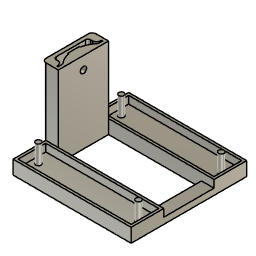
din_mount_cap_mcb_powerdist v2 (Autodesk Fusion 360 design; units mm, degrees)
Autodesk Fusion 360 part; units mm, degrees
note: some values were not read from the file. Set by a fixed rule: which sketch regions a step uses.
sketch "Sketch1" plane through (0, 0, 0) normal (0, 0, 1) x (1, 0, 0)
  line L0 (6.57, 33.77) -> (5.04, 33.77)
  line L1 (6.7574, 27.6038) -> (6.8807, 27.9464)
  arc A0 (5.5327, 24.59) -> (6.0311, 24.9915) centre (5.5327, 25.1) ccw
  arc A1 (10.1614, 33.4653) -> (6.8164, 27.7655) centre (24.5119, 21.2122) ccw
  line L2 (10.65, 34.79) -> (10.65, 37.85)
  line L3 (9.63, 3.17) -> (9.63, 2.15)
  arc A2 (6.0311, 15.0085) -> (6.8164, 12.2345) centre (28.9539, 20) ccw
  arc A3 (9.63, 3.17) -> (6.57, 6.23) centre (6.57, 3.17) ccw
  arc A4 (10.65, 5.21) -> (10.1614, 6.5347) centre (8.61, 5.21) ccw
  arc A5 (10.1614, 33.4653) -> (6.8164, 27.7655) centre (24.5119, 21.2122) ccw
  line L4 (5.1639, 24.59) -> (5.5327, 24.59)
  arc A6 (6.7574, 12.3962) -> (6.8164, 12.2345) centre (24.5119, 18.7878) ccw
  arc A7 (3, 8.27) -> (5.04, 6.23) centre (5.04, 8.27) ccw
  arc A8 (5.5327, 24.59) -> (6.0311, 24.9915) centre (5.5327, 25.1) ccw
  line L5 (11, 0) -> (11, 40)
  line L6 (0, 37) -> (0, 3)
  arc A9 (6.8164, 27.7655) -> (6.7574, 27.6038) centre (24.5119, 21.2122) ccw
  arc A10 (5.04, 33.77) -> (3, 31.73) centre (5.04, 31.73) ccw
  arc A11 (10.1614, 33.4653) -> (10.65, 34.79) centre (8.61, 34.79) ccw
  line L7 (6.8807, 12.0536) -> (6.7574, 12.3962)
  line L8 (3, 31.73) -> (3, 8.27)
  line L9 (3, 31.73) -> (3, 8.27)
  line L10 (5.1639, 15.41) -> (5.1639, 24.59)
  line L11 (5.1639, 15.41) -> (5.1639, 24.59)
  line L12 (6.8807, 12.0536) -> (6.7574, 12.3962)
  line L13 (10.65, 2.15) -> (10.65, 5.21)
  arc A12 (6.8807, 27.9464) -> (6.8164, 27.7655) centre (28.9539, 20) ccw
  line L14 (5.04, 6.23) -> (6.57, 6.23)
  line L15 (11, 40) -> (3, 40)
  line L16 (10.65, 2.15) -> (10.65, 5.21)
  line L17 (5.1639, 24.59) -> (5.5327, 24.59)
  arc A13 (6.7574, 12.3962) -> (6.8164, 12.2345) centre (24.5119, 18.7878) ccw
  line L18 (9.63, 3.17) -> (9.63, 2.15)
  line L19 (10.65, 37.85) -> (9.63, 37.85)
  arc A14 (6.8164, 12.2345) -> (10.1614, 6.5347) centre (24.5119, 18.7878) ccw
  line L20 (6.57, 33.77) -> (5.04, 33.77)
  line L21 (5.5327, 15.41) -> (5.1639, 15.41)
  arc A15 (6.0311, 15.0085) -> (5.5327, 15.41) centre (5.5327, 14.9) ccw
  arc A16 (3, 40) -> (0, 37) centre (3, 37) ccw
  line L22 (5.04, 6.23) -> (6.57, 6.23)
  line L23 (9.63, 37.85) -> (9.63, 36.83)
  arc A17 (6.8164, 27.7655) -> (6.0311, 24.9915) centre (28.9539, 20) ccw
  arc A18 (6.8164, 12.2345) -> (6.8807, 12.0536) centre (28.9539, 20) ccw
  arc A19 (10.1614, 33.4653) -> (10.65, 34.79) centre (8.61, 34.79) ccw
  arc A20 (5.04, 33.77) -> (3, 31.73) centre (5.04, 31.73) ccw
  line L24 (10.65, 34.79) -> (10.65, 37.85)
  line L25 (3, 0) -> (11, 0)
  line L26 (5.5327, 15.41) -> (5.1639, 15.41)
  arc A21 (0, 3) -> (3, 0) centre (3, 3) ccw
  arc A22 (6.0311, 15.0085) -> (5.5327, 15.41) centre (5.5327, 14.9) ccw
  arc A23 (10.65, 5.21) -> (10.1614, 6.5347) centre (8.61, 5.21) ccw
  line L27 (9.63, 2.15) -> (10.65, 2.15)
  line L28 (9.63, 37.85) -> (9.63, 36.83)
  arc A24 (6.8164, 27.7655) -> (6.0311, 24.9915) centre (28.9539, 20) ccw
  arc A25 (6.8807, 27.9464) -> (6.8164, 27.7655) centre (28.9539, 20) ccw
  arc A26 (6.8164, 12.2345) -> (6.8807, 12.0536) centre (28.9539, 20) ccw
  arc A27 (6.57, 33.77) -> (9.63, 36.83) centre (6.57, 36.83) ccw
  arc A28 (6.8164, 27.7655) -> (6.7574, 27.6038) centre (24.5119, 21.2122) ccw
  arc A29 (6.0311, 15.0085) -> (6.8164, 12.2345) centre (28.9539, 20) ccw
  arc A30 (6.57, 33.77) -> (9.63, 36.83) centre (6.57, 36.83) ccw
  line L29 (10.65, 37.85) -> (9.63, 37.85)
  line L30 (9.63, 2.15) -> (10.65, 2.15)
  arc A31 (9.63, 3.17) -> (6.57, 6.23) centre (6.57, 3.17) ccw
  arc A32 (3, 8.27) -> (5.04, 6.23) centre (5.04, 8.27) ccw
  line L31 (6.7574, 27.6038) -> (6.8807, 27.9464)
  arc A33 (6.8164, 12.2345) -> (10.1614, 6.5347) centre (24.5119, 18.7878) ccw
  line L32 (11, 40) -> (13, 40)
  line L33 (13, 40) -> (13, 0)
  line L34 (13, 0) -> (11, 0)
  line L35 (11, 0) -> (11, 40)
  point P0 (3, 20)
  point P1 (3, 20)
  point P2 (0, 40)
  dimension "d1" = 11
  dimension "d2" = 40
  dimension "d3" = 3
  dimension "d4" = 2
  dimension "d5" = 40
  constraint horizontal L25
  constraint vertical L5
  constraint horizontal L15
  constraint vertical L6
  constraint coincident P2 L15
  constraint coincident P2 L6
  constraint tangent L15 A16
  constraint tangent L6 A16
  constraint coincident origin L25
  constraint coincident origin L6
  constraint tangent L25 A21
  constraint tangent L6 A21
  constraint equal A16 A21
  constraint horizontal L32
  constraint vertical L33
  constraint horizontal L34
  constraint vertical L35
  measures "d1" distance of origin L5.start
  measures "d2" distance of origin P2
  measures "d3" radius of A16
  measures "d4" distance of L5.end L32.end
  measures "d5" distance of L5.end L5.start
extrude "Extrude1" add sketch "Sketch1" along normal blind 64.5
sketch "Sketch2" plane through (0, 0, 0) normal (-1, 0, 0) x (0, -1, 0)
  line L0 (-37, 0) -> (-3, 0)
  line L1 (-3, 0) -> (-3, 64.5)
  line L2 (-3, 64.5) -> (-37, 64.5)
  line L3 (-37, 64.5) -> (-37, 0)
  circle A0 centre (-20, 54.5) radius 2.5
  line L4 (0, 0) -> (0, 64.5)
  dimension "d8" = 5
  dimension "d9" = 10
  dimension "d10" = 20
  measures "d8" diameter of A0
  measures "d9" distance of L2 A0.centre
  measures "d10" distance of A0.centre L4
extrude "Extrude2" cut sketch "Sketch2" against normal blind 13 contours A0
sketch "Sketch3" plane through (0, 0, 0) normal (0, 0, -1) x (1, 0, 0)
  arc A0 (5.5327, -15.41) -> (6.0311, -15.0085) centre (5.5327, -14.9) ccw
  line L0 (5.5327, -15.41) -> (5.1639, -15.41)
  line L1 (5.1639, -15.41) -> (5.1639, -24.59)
  line L2 (5.1639, -24.59) -> (5.5327, -24.59)
  arc A1 (6.0311, -24.9915) -> (5.5327, -24.59) centre (5.5327, -25.1) ccw
  arc A2 (6.0311, -24.9915) -> (6.8164, -27.7655) centre (28.9539, -20) ccw
  arc A3 (6.8164, -27.7655) -> (10.1614, -33.4653) centre (24.5119, -21.2122) ccw
  arc A4 (10.65, -34.79) -> (10.1614, -33.4653) centre (8.61, -34.79) ccw
  line L3 (10.65, -34.79) -> (10.65, -37.85)
  line L4 (10.65, -37.85) -> (9.63, -37.85)
  line L5 (9.63, -37.85) -> (9.63, -36.83)
  arc A5 (9.63, -36.83) -> (6.57, -33.77) centre (6.57, -36.83) ccw
  line L6 (6.57, -33.77) -> (5.04, -33.77)
  arc A6 (3, -31.73) -> (5.04, -33.77) centre (5.04, -31.73) ccw
  line L7 (3, -31.73) -> (3, -8.27)
  arc A7 (5.04, -6.23) -> (3, -8.27) centre (5.04, -8.27) ccw
  line L8 (5.04, -6.23) -> (6.57, -6.23)
  arc A8 (6.57, -6.23) -> (9.63, -3.17) centre (6.57, -3.17) ccw
  line L9 (9.63, -3.17) -> (9.63, -2.15)
  line L10 (9.63, -2.15) -> (10.65, -2.15)
  line L11 (10.65, -2.15) -> (10.65, -5.21)
  arc A9 (10.1614, -6.5347) -> (10.65, -5.21) centre (8.61, -5.21) ccw
  arc A10 (10.1614, -6.5347) -> (6.8164, -12.2345) centre (24.5119, -18.7878) ccw
  arc A11 (6.8164, -12.2345) -> (6.0311, -15.0085) centre (28.9539, -20) ccw
  line L12 (3, -40) -> (13, -40)
  line L13 (13, -40) -> (13, 0)
  line L14 (13, 0) -> (3, 0)
  arc A12 (3, 0) -> (0, -3) centre (3, -3) ccw
  line L15 (0, -3) -> (0, -37)
  arc A13 (0, -37) -> (3, -40) centre (3, -37) ccw
  line L16 (3, -40) -> (97, -40)
  line L17 (97, -40) -> (97, -66)
  line L18 (97, -66) -> (3, -66)
  line L19 (3, -66) -> (3, -40)
  line L20 (3, 0) -> (97, 0)
  line L21 (97, 0) -> (97, 26)
  line L22 (97, 26) -> (3, 26)
  line L23 (3, 26) -> (3, 0)
  line L24 (97, -40) -> (87, -40)
  line L25 (87, -40) -> (87, 0)
  line L26 (87, 0) -> (97, 0)
  line L27 (97, 0) -> (97, -40)
  dimension "d13" = 94
  dimension "d14" = 26
  dimension "d15" = 94
  dimension "d16" = 26
  dimension "d17" = 10
  dimension "d18" = 40
  constraint horizontal L16
  constraint vertical L17
  constraint horizontal L18
  constraint vertical L19
  constraint coincident L12.start A13.end
  constraint horizontal L20
  constraint vertical L21
  constraint horizontal L22
  constraint vertical L23
  constraint coincident L14.end A12.start
  constraint horizontal L24
  constraint vertical L25
  constraint horizontal L26
  constraint vertical L27
  measures "d13" distance of L12.start L16.end
  measures "d14" distance of L12.start L18.end
  measures "d15" distance of L14.end L20.end
  measures "d16" distance of L14.end L22.end
  measures "d17" distance of L16.end L24.end
  measures "d18" distance of L16.end L20.end
extrude "Extrude3" add sketch "Sketch3" against normal blind 5 contours L12 L16 L17 L18 L19 L24 | L14 L20 L21 L22 L23 L26 | L16 L20 L24 L25 L26 L27
sketch "Sketch4" plane through (0, 0, 5) normal (0, 0, 1) x (-1, 0, 0)
  line L0 (-3, 26) -> (-97, 26)
  line L1 (-97, 26) -> (-97, -66)
  line L2 (-97, -66) -> (-3, -66)
  line L3 (-3, -66) -> (-3, -40)
  line L4 (-3, -40) -> (-13, -40)
  line L5 (-13, -40) -> (-87, -40)
  line L6 (-87, -40) -> (-87, 0)
  line L7 (-87, 0) -> (-13, 0)
  line L8 (-13, 0) -> (-3, 0)
  line L9 (-3, 0) -> (-3, 26)
  line L10 (-87, 0) -> (-97, 0)
  line L11 (-87, -40) -> (-97, -40)
  constraint coincident L6.end L7.start
  constraint coincident L1 L10.end
  constraint perpendicular L1 L10
  constraint coincident L5.end L6.start
  constraint coincident L1 L11.end
  constraint perpendicular L1 L11
extrude "Extrude4" add sketch "Sketch4" along normal blind 6 thin wall 2 inside contours L0 L1 L7 L8 L9 L10 | L1 L2 L3 L4 L5 L11
sketch "Sketch5" plane through (0, 0, 5) normal (0, 0, 1) x (-1, 0, 0)
  line L0 (-95, 24) -> (-95, 2)
  line L1 (-95, 2) -> (-5, 2)
  line L2 (-5, 2) -> (-5, 24)
  line L3 (-5, 24) -> (-95, 24)
  circle A0 centre (-10.15, 13) radius 2.15
  circle A1 centre (-89.85, 13) radius 2.15
  circle A2 centre (-10.15, -53) radius 2.15
  circle A3 centre (-89.85, -53) radius 2.15
  line L4 (-5, -64) -> (-95, -64)
  line L5 (-5, -42) -> (-5, -64)
  line L6 (-95, -64) -> (-95, -42)
  dimension "d24" = 4.3
  dimension "d25" = 11
  dimension "d26" = 5.15
  dimension "d27" = 4.3
  dimension "d28" = 5.15
  dimension "d29" = 11
  dimension "d30" = 4.3
  dimension "d31" = 4.3
  dimension "d32" = 11
  dimension "d33" = 5.15
  dimension "d34" = 5.15
  dimension "d35" = 11
  measures "d24" diameter of A0
  measures "d25" distance of L3 A0.centre
  measures "d26" distance of L2 A0.centre
  measures "d27" diameter of A1
  measures "d28" distance of L0 A1.centre
  measures "d29" distance of L3 A1.centre
  measures "d30" diameter of A2
  measures "d31" diameter of A3
  measures "d32" distance of A2.centre L4
  measures "d33" distance of A2.centre L5
  measures "d34" distance of A3.centre L6
  measures "d35" distance of A3.centre L4
extrude "Extrude5" add sketch "Sketch5" along normal blind 15 contours A0 | A1 | A2 | A3
